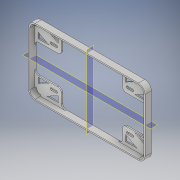
# Autodesk Inventor part: Hub Enclosure Front (new)
Saved by Autodesk Inventor 2018 (Build 220112000, 112)
## iProperties
Created: 2018-03-26
Part Number: Hub Enclosure Front (new)
Material: Generic
Document SubType Name: Modeling
Designer: brutu
Density: 1 g/cm^3
Appearance: Default
Author: brutu
Autodesk Inventor part; units mm, degrees
ref_plane "YZ Plane" through (0, 0, 0) normal (1, 0, 0) x (0, 1, 0)
ref_plane "XZ Plane" through (0, 0, 0) normal (0, 1, 0) x (-1, 0, 0)
ref_plane "XY Plane" through (0, 0, 0) normal (0, 0, 1) x (1, 0, 0)
sketch "Sketch1" plane through (0, 0, 0) normal (0, 0, 1) x (1, 0, 0)
  arc A0 (0, -0.381) -> (11, 10.619) centre (0, 10.619) ccw projected
  line L0 (11, 99.379) -> (11, 10.619) projected
  line L1 (0, -0.381) -> (-170.96, -0.381) projected
  arc A1 (11, 99.379) -> (0, 110.379) centre (0, 99.379) ccw projected
  line L2 (-170.96, 110.379) -> (0, 110.379) projected
  arc A2 (-170.96, 110.379) -> (-181.96, 99.379) centre (-170.96, 99.379) ccw projected
  line L3 (-181.96, 10.619) -> (-181.96, 99.379) projected
  arc A3 (-181.96, 10.619) -> (-170.96, -0.381) centre (-170.96, 10.619) ccw projected
  circle A4 centre (-22.38, 21.199) radius 1.5 projected
  circle A5 centre (-148.58, 21.199) radius 1.5 projected
  circle A6 centre (-148.58, 86.849) radius 1.5 projected
  circle A7 centre (-22.38, 86.849) radius 1.5 projected
  circle A8 centre (-22.38, 21.199) radius 1.905
  circle A9 centre (-22.38, 86.849) radius 1.905
  line L4 (-41.31, 1.719) -> (-129.65, 1.719)
  line L5 (-129.65, 108.279) -> (-41.31, 108.279)
  line L6 (8.9, 71.419) -> (8.9, 36.009)
  line L7 (-34.96, 23.309) -> (-34.96, 8.069)
  line L8 (-28.61, 29.659) -> (2.55, 29.659)
  arc A10 (-28.61, 29.659) -> (-34.96, 23.309) centre (-28.61, 23.309) ccw
  line L9 (2.55, 77.769) -> (-28.61, 77.769)
  line L10 (-34.96, 84.119) -> (-34.96, 101.929)
  arc A11 (-34.96, 84.119) -> (-28.61, 77.769) centre (-28.61, 84.119) ccw
  arc A12 (2.55, 29.659) -> (8.9, 36.009) centre (2.55, 36.009) ccw
  arc A13 (-41.31, 1.719) -> (-34.96, 8.069) centre (-41.31, 8.069) ccw
  arc A14 (-34.96, 101.929) -> (-41.31, 108.279) centre (-41.31, 101.929) ccw
  arc A15 (8.9, 71.419) -> (2.55, 77.769) centre (2.55, 71.419) ccw
  line L11 (-29.88, 25.199) -> (-29.88, 17.199) projected
  line L12 (-14.88, 25.199) -> (-29.88, 25.199) projected
  line L13 (-29.88, 82.849) -> (-14.88, 82.849) projected
  line L14 (-29.88, 90.849) -> (-29.88, 82.849) projected
  circle A16 centre (-148.58, 21.199) radius 1.905
  circle A17 centre (-148.58, 86.849) radius 1.905
  line L15 (-179.86, 71.419) -> (-179.86, 36.009)
  line L16 (-136, 23.309) -> (-136, 8.069)
  line L17 (-142.35, 29.659) -> (-173.51, 29.659)
  arc A18 (-136, 23.309) -> (-142.35, 29.659) centre (-142.35, 23.309) ccw
  line L18 (-173.51, 77.769) -> (-142.35, 77.769)
  line L19 (-136, 84.119) -> (-136, 101.929)
  arc A19 (-142.35, 77.769) -> (-136, 84.119) centre (-142.35, 84.119) ccw
  arc A20 (-179.86, 36.009) -> (-173.51, 29.659) centre (-173.51, 36.009) ccw
  arc A21 (-136, 8.069) -> (-129.65, 1.719) centre (-129.65, 8.069) ccw
  arc A22 (-129.65, 108.279) -> (-136, 101.929) centre (-129.65, 101.929) ccw
  arc A23 (-173.51, 77.769) -> (-179.86, 71.419) centre (-173.51, 71.419) ccw
  point P0 (0, 0)
  point P1 (-34.96, 1.719)
  point P2 (8.9, 29.659)
  point P3 (8.9, 77.769)
  point P4 (-34.96, 77.769)
  point P5 (-34.96, 108.279)
  dimension "d1" = 23.53
  dimension "d2" = 3.81
  dimension "d5" = 3.81
  dimension "d16" = 27.94
  dimension "d18" = 6.35
  dimension "d21" = 6.35
  dimension "d22" = 6.35
  dimension "d23" = 2.1
  dimension "d24" = 2.1
  dimension "d25" = 2.1
  dimension "d33" = 5.08
  dimension "d34" = 5.08
  dimension "d35" = 5.08
  dimension "d36" = 6.35
  dimension "d37" = 6.35
  constraints: 25 point on circle, 24 end point, 16 centre point, 12 tangent, 10 point on line, 2 coincident, 2 perpendicular, 1 equal radius, 1 horizontal, 1 vertical
  measures "d1" distance from line of L2 A7.centre
  measures "d2" diameter of A8
  measures "d5" diameter of A9
  measures "d16" distance between parallel lines of L4 L8
  measures "d18" radius of A10
  measures "d21" radius of A11
  measures "d22" radius of A12
  measures "d23" distance between parallel lines of L1 L4
  measures "d24" distance between parallel lines of L0 L6
  measures "d25" distance between parallel lines of L2 L5
  measures "d33" distance between parallel lines of L9 L13
  measures "d34" distance between parallel lines of L7 L11
  measures "d35" distance between parallel lines of L10 L14
  measures "d36" radius of A14
  measures "d37" radius of A15
extrude "Extrusion3" add sketch "Sketch1" along normal blind 2.1 contours L1 A3 L3 A2 L2 A1 L0 A0
sketch "Sketch4" plane through (0, 0, 2.1) normal (0, 0, 1) x (1, 0, 0)
  arc A0 (-28.61, 29.659) -> (-34.96, 23.309) centre (-28.61, 23.309) ccw projected
  line L0 (-34.96, 23.309) -> (-34.96, 8.069) projected
  arc A1 (-41.31, 1.719) -> (-34.96, 8.069) centre (-41.31, 8.069) ccw projected
  line L1 (-41.31, 1.719) -> (-129.65, 1.719) projected
  arc A2 (-136, 8.069) -> (-129.65, 1.719) centre (-129.65, 8.069) ccw projected
  line L2 (-136, 8.069) -> (-136, 23.309) projected
  arc A3 (-136, 23.309) -> (-142.35, 29.659) centre (-142.35, 23.309) ccw projected
  line L3 (-142.35, 29.659) -> (-173.51, 29.659) projected
  arc A4 (-179.86, 36.009) -> (-173.51, 29.659) centre (-173.51, 36.009) ccw projected
  line L4 (-179.86, 36.009) -> (-179.86, 71.419) projected
  arc A5 (-173.51, 77.769) -> (-179.86, 71.419) centre (-173.51, 71.419) ccw projected
  line L5 (-173.51, 77.769) -> (-142.35, 77.769) projected
  arc A6 (-142.35, 77.769) -> (-136, 84.119) centre (-142.35, 84.119) ccw projected
  line L6 (-136, 84.119) -> (-136, 101.929) projected
  arc A7 (-129.65, 108.279) -> (-136, 101.929) centre (-129.65, 101.929) ccw projected
  line L7 (-129.65, 108.279) -> (-41.31, 108.279) projected
  arc A8 (-34.96, 101.929) -> (-41.31, 108.279) centre (-41.31, 101.929) ccw projected
  line L8 (-34.96, 101.929) -> (-34.96, 84.119) projected
  arc A9 (-34.96, 84.119) -> (-28.61, 77.769) centre (-28.61, 84.119) ccw projected
  line L9 (-28.61, 77.769) -> (2.55, 77.769) projected
  arc A10 (8.9, 71.419) -> (2.55, 77.769) centre (2.55, 71.419) ccw projected
  line L10 (8.9, 71.419) -> (8.9, 36.009) projected
  arc A11 (2.55, 29.659) -> (8.9, 36.009) centre (2.55, 36.009) ccw projected
  line L11 (2.55, 29.659) -> (-28.61, 29.659) projected
  circle A12 centre (-148.58, 86.849) radius 1.905 projected
  circle A13 centre (-148.58, 21.199) radius 1.905 projected
  circle A14 centre (-22.38, 86.849) radius 1.905 projected
  circle A15 centre (-22.38, 21.199) radius 1.905 projected
  arc A16 (0, -0.381) -> (11, 10.619) centre (0, 10.619) ccw projected
  line L12 (11, 10.619) -> (11, 99.379) projected
  arc A17 (11, 99.379) -> (0, 110.379) centre (0, 99.379) ccw projected
  line L13 (0, 110.379) -> (-170.96, 110.379) projected
  arc A18 (-170.96, 110.379) -> (-181.96, 99.379) centre (-170.96, 99.379) ccw projected
  line L14 (-181.96, 99.379) -> (-181.96, 10.619) projected
  arc A19 (-181.96, 10.619) -> (-170.96, -0.381) centre (-170.96, 10.619) ccw projected
  line L15 (-170.96, -0.381) -> (0, -0.381) projected
  arc A20 (0, 1.719) -> (8.9, 10.619) centre (0, 10.619) ccw
  line L16 (8.9, 10.619) -> (8.9, 99.379)
  arc A21 (8.9, 99.379) -> (0, 108.279) centre (0, 99.379) ccw
  line L17 (0, 108.279) -> (-170.96, 108.279)
  arc A22 (-170.96, 108.279) -> (-179.86, 99.379) centre (-170.96, 99.379) ccw
  line L18 (-179.86, 99.379) -> (-179.86, 10.619)
  arc A23 (-179.86, 10.619) -> (-170.96, 1.719) centre (-170.96, 10.619) ccw
  line L19 (-170.96, 1.719) -> (0, 1.719)
  point P0 (0, 0)
  dimension "d40" = 2.1
  constraints: 8 end point, 8 point on circle, 4 centre point, 7 other
  measures "d40" distance between parallel lines of L15 L19
extrude "Extrusion4" add sketch "Sketch4" along normal blind 8.5 contours L15 A19 L14 A18 L13 A17 L12 A16
ref_plane "Work Plane1" through (-85.48, 10.619, 10.6) normal (-1, 0, 0) x (0, 0, 1)
ref_plane "Work Plane2" through (-170.96, 54.999, 10.6) normal (0, -1, 0) x (1, 0, 0)
sketch "Sketch9" plane through (0, 0, 0) normal (0, 0, -1) x (-1, 0, 0)
  arc A0 (-8.9, 10.619) -> (0, 1.719) centre (0, 10.619) ccw projected
  arc A1 (-6.8, 10.619) -> (0, 3.819) centre (0, 10.619) ccw projected
  line L0 (0, 1.719) -> (0, 3.819) projected
  line L1 (-6.8, 10.619) -> (-8.9, 10.619) projected
  arc A2 (170.96, 1.719) -> (179.86, 10.619) centre (170.96, 10.619) ccw projected
  arc A3 (170.96, 3.819) -> (177.76, 10.619) centre (170.96, 10.619) ccw projected
  line L2 (170.96, 3.819) -> (170.96, 1.719) projected
  line L3 (179.86, 10.619) -> (177.76, 10.619) projected
  arc A4 (179.86, 99.379) -> (170.96, 108.279) centre (170.96, 99.379) ccw projected
  arc A5 (177.76, 99.379) -> (170.96, 106.179) centre (170.96, 99.379) ccw projected
  line L4 (177.76, 99.379) -> (179.86, 99.379) projected
  line L5 (170.96, 108.279) -> (170.96, 106.179) projected
  arc A6 (0, 106.179) -> (-6.8, 99.379) centre (0, 99.379) ccw projected
  arc A7 (0, 108.279) -> (-8.9, 99.379) centre (0, 99.379) ccw projected
  line L6 (-8.9, 99.379) -> (-6.8, 99.379) projected
  line L7 (0, 106.179) -> (0, 108.279) projected
  line L8 (170.96, 1.719) -> (0, 1.719) projected
  line L9 (0.508, 1.719) -> (0, 1.719)
  line L10 (-6.36, 11.127) -> (-8.9, 11.127)
  line L11 (-8.9, 11.127) -> (-8.9, 10.619)
  line L12 (0.508, 1.719) -> (0.508, 4.259)
  arc A8 (-6.36, 11.127) -> (0.508, 4.259) centre (0.748, 11.367) ccw
  arc A9 (-8.9, 10.619) -> (0, 1.719) centre (0, 10.619) ccw
  line L13 (-6.36, 98.871) -> (-8.9, 98.871)
  line L14 (-8.9, 99.379) -> (-8.9, 10.619) projected
  line L15 (0.508, 105.739) -> (0.508, 108.279)
  line L16 (0.508, 108.279) -> (0, 108.279)
  arc A10 (0, 108.279) -> (-8.9, 98.871) centre (0, 99.3653) ccw
  arc A11 (0.508, 105.739) -> (-6.36, 98.871) centre (0.748, 98.631) ccw
  line L17 (0, -0.381) -> (170.96, -0.381) projected
  line L18 (85.48, -0.381) -> (85.48, 110.379)
  line L19 (170.96, 110.379) -> (0, 110.379) projected
  arc A12 (170.96, 1.719) -> (179.86, 10.619) centre (170.96, 10.619) ccw
  line L20 (170.452, 1.719) -> (170.96, 1.719)
  line L21 (177.32, 11.127) -> (179.86, 11.127)
  line L22 (170.452, 1.719) -> (170.452, 4.259)
  arc A13 (170.452, 4.259) -> (177.32, 11.127) centre (170.212, 11.367) ccw
  line L23 (177.32, 98.871) -> (179.86, 98.871)
  line L24 (179.86, 99.379) -> (179.86, 10.619)
  line L25 (170.452, 105.739) -> (170.452, 108.279)
  line L26 (170.452, 108.279) -> (170.96, 108.279)
  arc A14 (179.86, 98.871) -> (170.96, 108.279) centre (170.96, 99.3653) ccw
  arc A15 (177.32, 98.871) -> (170.452, 105.739) centre (170.212, 98.631) ccw
  point P0 (0, 0)
  point P1 (17.526, 1.719)
  dimension "d73" = 0.508
  dimension "d74" = 0.508
  dimension "d75" = 2.54
  dimension "d76" = 2.54
  dimension "d77" = 7.112
  dimension "d78" = 2.54
  dimension "d79" = 2.54
  dimension "d80" = 0.508
  dimension "d81" = 0.508
  dimension "d82" = 7.112
  constraints: 30 end point, 16 point on circle, 12 symmetric about line, 8 centre point, 3 horizontal, 2 midpoint, 2 perpendicular, 2 point on line, 2 vertical, 1 concentric, 1 tangent, 4 other
  measures "d73" distance between parallel lines of L0 L12
  measures "d74" distance between parallel lines of L1 L10
  measures "d75" horizontal distance of L10.start L1.end
  measures "d76" distance of L9.start L12.end
  measures "d77" radius of A8
  measures "d78" distance of L13.start L13.end
  measures "d79" distance of L15.start L15.end
  measures "d80" distance of L15.end L7.end
  measures "d81" distance between parallel lines of L13 L6
  measures "d82" radius of A11
extrude "Extrusion7" cut sketch "Sketch9" against normal up to next contours L1 A1 L0 A0 | L7 A6 L6 A7 | A10 L16 L15 A11 L13 | L23 A15 L25 L26 L5 A5 L4 L24 | L24 A4 A14 | L22 A13 L21 L24 L3 A3 L2 L8 | L2 A3 L3 A2 | L4 A5 L5 A4
sketch "Sketch10" plane through (0, 0, 0) normal (0, 0, -1) x (-1, 0, 0)
  line L0 (-3.38, 18.0763) -> (14.4, 27.559)
  line L1 (14.4, 27.559) -> (-3.38, 27.559)
  line L2 (-3.38, 27.559) -> (-3.38, 18.0763)
  line L3 (10.7529, 7.239) -> (29.8029, 17.399)
  line L4 (29.8029, 17.399) -> (29.8029, 7.239)
  line L5 (29.8029, 7.239) -> (10.7529, 7.239)
  line L6 (0, -0.381) -> (170.96, -0.381) projected
  line L7 (-11, 99.379) -> (-11, 10.619) projected
  line L8 (181.96, 99.379) -> (181.96, 10.619) projected
  line L9 (181.96, 54.999) -> (-11, 54.999)
  line L10 (-11, 10.619) -> (-11, 99.379) projected
  line L11 (85.48, -0.381) -> (85.48, 110.379)
  line L12 (0, 110.379) -> (170.96, 110.379) projected
  line L13 (174.34, 18.0763) -> (156.56, 27.559)
  line L14 (156.56, 27.559) -> (174.34, 27.559)
  line L15 (174.34, 27.559) -> (174.34, 18.0763)
  line L16 (160.2071, 7.239) -> (141.1571, 17.399)
  line L17 (141.1571, 17.399) -> (141.1571, 7.239)
  line L18 (141.1571, 7.239) -> (160.2071, 7.239)
  line L19 (-3.38, 91.9217) -> (14.4, 82.439)
  line L20 (14.4, 82.439) -> (-3.38, 82.439)
  line L21 (-3.38, 82.439) -> (-3.38, 91.9217)
  line L22 (10.7529, 102.759) -> (29.8029, 92.599)
  line L23 (29.8029, 92.599) -> (29.8029, 102.759)
  line L24 (29.8029, 102.759) -> (10.7529, 102.759)
  line L25 (141.1571, 102.759) -> (160.2071, 102.759)
  line L26 (141.1571, 92.599) -> (141.1571, 102.759)
  line L27 (160.2071, 102.759) -> (141.1571, 92.599)
  line L28 (174.34, 91.9217) -> (156.56, 82.439)
  line L29 (156.56, 82.439) -> (174.34, 82.439)
  line L30 (174.34, 82.439) -> (174.34, 91.9217)
  point P0 (0, 0)
  point P1 (-11, 19.255)
  dimension "d85" = 17.78
  dimension "d86" = 19.05
  dimension "d87" = 10.16
  dimension "d88" = 7.62
  dimension "d89" = 7.62
  dimension "d102" = 27.94
  constraints: 52 end point, 18 symmetric about line, 4 midpoint, 2 parallel, 2 perpendicular, 1 horizontal
  measures "d85" distance of L0.end L1.end
  measures "d86" distance of L4.end L3.start
  measures "d87" distance of L3.end L4.end
  measures "d88" distance between parallel lines of L6 L5
  measures "d89" distance between parallel lines of L7 L2
  measures "d102" distance between parallel lines of L6 L1
extrude "Extrusion8" cut sketch "Sketch10" against normal up to next
sketch "Sketch11" plane through (0, 0, 2.1) normal (0, 0, 1) x (1, 0, 0)
  arc A0 (-144.389, 84.944) -> (-144.389, 88.754) centre (-144.389, 86.849) ccw
  circle A1 centre (-148.58, 86.849) radius 1.905 projected
  arc A2 (-152.771, 88.754) -> (-152.771, 84.944) centre (-152.771, 86.849) ccw
  line L0 (-152.771, 88.754) -> (-144.389, 88.754)
  line L1 (-144.389, 84.944) -> (-152.771, 84.944)
  circle A3 centre (-148.58, 21.199) radius 1.905 projected
  arc A4 (-144.389, 19.294) -> (-144.389, 23.104) centre (-144.389, 21.199) ccw
  arc A5 (-152.771, 23.104) -> (-152.771, 19.294) centre (-152.771, 21.199) ccw
  line L2 (-152.771, 23.104) -> (-144.389, 23.104)
  line L3 (-152.771, 19.294) -> (-144.389, 19.294)
  line L4 (-85.48, -22.533) -> (-85.48, 132.531) projected
  arc A6 (-26.571, 88.754) -> (-26.571, 84.944) centre (-26.571, 86.849) ccw
  arc A7 (-18.189, 84.944) -> (-18.189, 88.754) centre (-18.189, 86.849) ccw
  line L5 (-18.189, 88.754) -> (-26.571, 88.754)
  line L6 (-26.571, 84.944) -> (-18.189, 84.944)
  arc A8 (-26.571, 23.104) -> (-26.571, 19.294) centre (-26.571, 21.199) ccw
  arc A9 (-18.189, 19.294) -> (-18.189, 23.104) centre (-18.189, 21.199) ccw
  line L7 (-18.189, 23.104) -> (-26.571, 23.104)
  line L8 (-18.189, 19.294) -> (-26.571, 19.294)
  point P0 (0, 0)
  point P1 (-148.58, 88.754)
  point P2 (-148.58, 23.104)
  dimension "d92" = 3.81
  dimension "d93" = 1.905
  dimension "d94" = 1.905
  dimension "d96" = 8.382
  dimension "d97" = 1.905
  dimension "d98" = 1.905
  dimension "d101" = 8.382
  constraints: 16 end point, 16 point on circle, 12 symmetric about line, 8 centre point, 7 vertical alignment, 3 horizontal, 2 midpoint, 2 tangent, 1 parallel, 4 other
  measures "d92" diameter of A1
  measures "d93" radius of A0
  measures "d94" radius of A2
  measures "d96" distance of L1.start L1.end
  measures "d97" radius of A4
  measures "d98" radius of A5
  measures "d101" distance of L2.start L2.end
extrude "Extrusion9" cut sketch "Sketch11" against normal up to next contours L1 A1 L0 A0 | L1 A2 L0 A1 | A3 L2 A4 L3 | A3 L3 A5 L2 | L5 A7 L6 A6 | L7 A9 L8 A8
equation "\"d24\" = d23"
equation "\"d25\" = d23"
equation "\"d36\" = d22"
equation "\"d37\" = d22"
equation "\"d74\" = d73"
equation "\"d76\" = d75"
equation "\"d78\" = d75"
equation "\"d79\" = d78"
equation "\"d80\" = d74"
equation "\"d81\" = d80"
equation "\"d82\" = d77"
equation "\"d93\" = 0.5 * d92"
equation "\"d94\" = 0.5 * d95"
equation "\"d97\" = d93"
equation "\"d98\" = d99"
equation "\"d101\" = d96"
equation "\"d99\" = 0.5 * d100"
equation "\"d95\" = 3.81"
equation "\"d100\" = 3.81"
body "Solid2"
